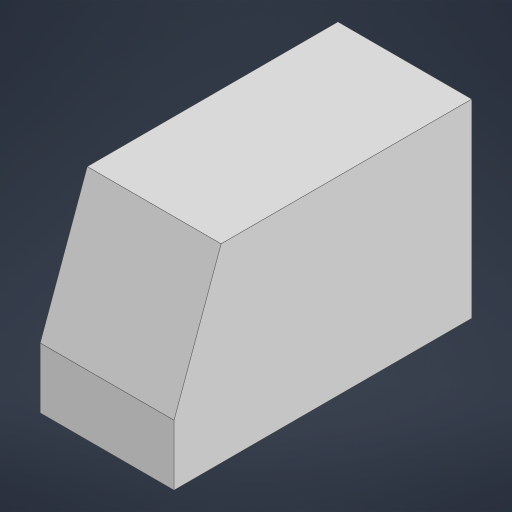
# Autodesk Inventor part: Electronics Case for Bubba
Saved by Autodesk Inventor 2024 (Build 280153000, 153)
## iProperties
Created: 2025-04-03
Part Number: Electronics Case for Bubba
Material: Generic
Document SubType Name: Modeling
Designer: Vincent Larson
Density: 1 g/cm^3
Appearance: Default
Author: Vincent Larson
Autodesk Inventor part; units mm, degrees
ref_plane "YZ Plane" through (0, 0, 0) normal (1, 0, 0) x (0, 1, 0)
ref_plane "XZ Plane" through (0, 0, 0) normal (0, 1, 0) x (-1, 0, 0)
ref_plane "XY Plane" through (0, 0, 0) normal (0, 0, 1) x (1, 0, 0)
sketch "Sketch1" plane through (0, 0, 0) normal (1, 0, 0) x (0, 1, 0)
  line L0 (0, 0) -> (171.45, 0)
  line L1 (171.45, 0) -> (171.45, -271.78)
  line L2 (171.45, -271.78) -> (0, -271.78)
  line L3 (0, -271.78) -> (0, 0)
  line L4 (0, 0) -> (53.34, 0)
  line L5 (53.34, 0) -> (53.34, -271.78)
  line L6 (53.34, 0) -> (171.45, -42.9885)
  line L7 (53.34, 0) -> (179.03, 0) construction
  line L8 (173.99, -274.32) -> (173.99, 2.54)
  line L9 (173.99, 2.54) -> (-2.54, 2.54)
  line L10 (-2.54, 2.54) -> (-2.54, -274.32)
  line L11 (-2.54, -274.32) -> (173.99, -274.32)
  line L12 (54.2087, 2.3868) -> (172.3187, -40.6017)
  line L13 (179.03, -43.0444) -> (43.4558, 6.3006)
  point P0 (53.7879, 2.54)
  point P1 (173.99, -41.21)
  dimension "d0" = 171.45
  dimension "d1" = 271.78
  dimension "d2" = 53.34
  dimension "d3" = 20
  dimension "d4" = 2.54
  dimension "d5" = 2.54
  constraints: 28 end point, 5 parallel, 5 point on line, 3 perpendicular, 2 horizontal, 1 equal length, 3 other
  measures "d0" distance of L1.end L2.end
  measures "d1" distance of L0.end L1.end
  measures "d2" distance of L0.start L4.end
  measures "d3" angle of L6 L7
  measures "d4" distance between parallel lines of L1 L8
  measures "d5" distance between parallel lines of L6 L12
extrude "Extrusion1" add sketch "Sketch1" along normal blind 121.92 contours L3 L2 L1 L12 L13 L8 L11 L10 L9 L0 | L0 L12 L1 L6
sketch "Sketch2" plane through (121.92, 0, 0) normal (1, 0, 0) x (0, 0, -1)
  line L0 (0, 0) -> (0, 53.34) projected
  line L1 (0, 53.34) -> (271.78, 53.34)
  line L2 (271.78, 171.45) -> (271.78, 0) projected
  line L3 (271.78, 55.88) -> (-2.54, 55.88)
  line L4 (-2.54, 55.88) -> (-2.54, 0)
  line L5 (0, 53.34) -> (42.9885, 171.45) projected
  line L6 (5.0738, 67.2802) -> (-1.6206, 48.8875)
  line L7 (271.78, 82.1996) -> (271.78, 27.94)
  point P0 (0.9245, 55.88)
  dimension "d8" = 2.54
  constraints: 10 end point, 4 point on line, 1 collinear, 1 horizontal, 1 other
  measures "d8" distance between parallel lines of L1 L3
extrude "Extrusion2" add sketch "Sketch2" against normal blind 121.92
sketch "Sketch3" plane through (0, -2.54, -274.32) normal (0, 0, -1) x (-1, 0, 0)
  line L0 (0, 0) -> (-121.92, 0) projected
  line L1 (-121.92, 0) -> (0, 0)
  line L2 (-121.92, 55.88) -> (0, 55.88) projected
  line L3 (0, 0) -> (0, 55.88)
  line L4 (0, 55.88) -> (-121.92, 55.88)
  line L5 (0, 58.42) -> (-121.92, 58.42) projected
  line L6 (-121.92, 55.88) -> (-121.92, 0)
  circle A0 centre (-60.96, 27.94) radius 27.94
  line L7 (-83.46, 13.94) -> (-38.46, 13.94)
  line L8 (-38.46, 13.94) -> (-38.46, 41.94)
  line L9 (-38.46, 41.94) -> (-83.46, 41.94)
  line L10 (-83.46, 41.94) -> (-83.46, 13.94)
  line L11 (-83.46, 13.94) -> (-38.46, 41.94) construction
  line L12 (-38.46, 13.94) -> (-83.46, 41.94) construction
  line L13 (-60.9761, 7.94) -> (-60.9439, 7.94)
  line L14 (-60.9439, 47.94) -> (-60.9761, 47.94)
  line L15 (-60.9761, 7.94) -> (-60.9439, 47.94) construction
  line L16 (-60.9439, 7.94) -> (-60.9761, 47.94) construction
  circle A1 centre (-60.96, 47.94) radius 1.8
  circle A2 centre (-60.96, 7.94) radius 1.8
  line L17 (-60.9761, 47.94) -> (-60.9761, 46.1401)
  line L18 (-60.9439, 46.1401) -> (-60.9439, 47.94)
  line L19 (-60.9761, 41.94) -> (-60.9761, 13.94)
  line L20 (-60.9761, 9.7399) -> (-60.9761, 7.94)
  line L21 (-60.9439, 7.94) -> (-60.9439, 9.7399)
  line L22 (-60.9439, 13.94) -> (-60.9439, 41.94)
  point P0 (0, 2.54)
  dimension "d11" = 45
  dimension "d12" = 28
  dimension "d13" = 40
  dimension "d14" = 3.6
  constraints: 40 end point, 13 parallel, 6 midpoint, 6 perpendicular, 4 point on circle, 4 point on line, 3 centre point, 3 horizontal
  measures "d11" distance of L9.end L8.end
  measures "d12" distance of L8.end L7.end
  measures "d13" distance of L14.start L13.end
  measures "d14" diameter of A1
extrude "Extrusion3" cut sketch "Sketch3" against normal blind 121.92 contours L10 L9 L19 L7 | L19 L9 L22 L7 | L22 L9 L8 L7 | L20 A2 L21 L13 | L13 L21 A2 L20 | L18 A1 L17 L14 | L14 L17 A1 L18
sketch "Sketch4" plane through (0, -2.54, -274.32) normal (0, 0, -1) x (-1, 0, 0)
  line L0 (-38.46, 41.94) -> (-38.46, 13.94) projected
  line L1 (-83.46, 13.94) -> (-83.46, 41.94) projected
  line L2 (-38.46, 41.94) -> (-83.46, 41.94)
  line L3 (-83.46, 41.94) -> (-83.46, 13.94)
  line L4 (-83.46, 13.94) -> (-38.46, 13.94)
  line L5 (-38.46, 13.94) -> (-38.46, 41.94)
  line L6 (-86.36, 13.94) -> (-35.56, 13.94)
  line L7 (-35.56, 13.94) -> (-35.56, 41.94)
  line L8 (-35.56, 41.94) -> (-86.36, 41.94)
  line L9 (-86.36, 41.94) -> (-86.36, 13.94)
  line L10 (-86.36, 13.94) -> (-35.56, 41.94) construction
  line L11 (-35.56, 13.94) -> (-86.36, 41.94) construction
  point P0 (0, 2.54)
  point P1 (-60.96, 27.94)
  dimension "d17" = 50.8
  constraints: 20 end point, 4 parallel, 2 horizontal, 2 midpoint, 2 perpendicular
  measures "d17" distance of L8.end L7.end
extrude "Extrusion4" cut sketch "Sketch4" against normal blind 121.92 contours L8 L7 L6 L0 | L1 L6 L9 L8
sketch "Sketch5" plane through (121.92, 0, 0) normal (1, 0, 0) x (0, 0, -1)
  line L0 (271.78, 53.34) -> (271.78, 0) projected
  line L1 (271.78, 53.34) -> (246.38, 53.34)
  line L2 (271.78, 53.34) -> (0, 53.34) projected
  line L3 (246.38, 53.34) -> (246.38, 43.18)
  line L4 (246.38, 43.18) -> (272.1958, 43.18)
  line L5 (246.38, 43.18) -> (226.8063, 53.34)
  line L6 (226.8063, 53.34) -> (209.4202, 62.3644)
  line L7 (245.2098, 40.9256) -> (225.6361, 51.0856)
  line L8 (225.6361, 51.0856) -> (208.25, 60.1101)
  line L9 (246.38, 40.64) -> (272.1958, 40.64)
  line L10 (239.3965, 43.9431) -> (259.2879, 33.6182)
  line L11 (267.1647, 40.64) -> (232.6379, 40.64)
  point P0 (0, 0)
  point P1 (245.7601, 40.64)
  point P2 (271.78, 40.64)
  point P3 (271.78, 43.18)
  point P4 (221.2929, 53.34)
  dimension "d20" = 25.4
  dimension "d21" = 10.16
  dimension "d22" = 2.54
  dimension "d23" = 2.54
  constraints: 20 end point, 7 point on line, 1 parallel, 1 perpendicular, 1 vertical, 1 other
  measures "d20" distance of L0.start L1.end
  measures "d21" distance of L1.end L3.end
  measures "d22" distance between parallel lines of L5 L7
  measures "d23" distance between parallel lines of L4 L9
extrude "Extrusion5" add sketch "Sketch5" against normal blind 121.92 contours L0 L9 L11 L10 L7 L8 L2 L5 L4
sketch "Sketch6" plane through (0, 0, 0) normal (-1, 0, 0) x (0, 0, 1)
  line L0 (-226.8063, 53.34) -> (-246.38, 43.18) projected
  line L1 (-233.7398, 49.741) -> (-197.786, 68.4033)
  line L2 (-197.786, 68.4033) -> (-271.78, 69.3117)
  line L3 (-271.78, 171.45) -> (-271.78, 55.88) projected
  line L4 (-271.78, 69.3117) -> (-271.78, 47.3341)
  line L5 (-271.78, 53.34) -> (-271.78, 43.18) projected
  line L6 (-271.78, 47.3341) -> (-233.7398, 49.741)
  point P0 (0, 0)
  constraints: 8 end point, 3 point on line, 1 collinear
extrude "Extrusion6" cut sketch "Sketch6" against normal blind 121.92
sketch "Sketch7" plane through (121.92, 0, 0) normal (1, 0, 0) x (0, 0, -1)
  line L0 (-2.54, -2.54) -> (274.32, -2.54) projected
  line L1 (274.32, 173.99) -> (41.21, 173.99) projected
  line L2 (-2.54, -2.54) -> (274.32, -2.54)
  line L3 (274.32, -2.54) -> (274.32, 173.99)
  line L4 (274.32, 173.99) -> (-2.54, 173.99)
  line L5 (-2.54, 173.99) -> (-2.54, -2.54)
  line L6 (41.21, 173.99) -> (-2.54, 53.7879) projected
  line L7 (41.21, 173.99) -> (-2.54, 53.7879)
  point P0 (0, 0)
  constraints: 10 end point, 3 equal length, 1 horizontal, 1 perpendicular
extrude "Extrusion7" add sketch "Sketch7" along normal blind 2.54 contours L5 L6 L1 L3 L0
sketch "Sketch8" plane through (0, -2.54, -274.32) normal (0, 0, -1) x (-1, 0, 0)
  line L0 (0, 173.99) -> (-121.92, 173.99) projected
  line L1 (-121.92, 173.99) -> (0, 173.99)
  line L2 (0, 173.99) -> (0, 52.07)
  line L3 (0, 52.07) -> (-121.92, 52.07)
  line L4 (-121.92, 52.07) -> (-121.92, 173.99)
  circle A0 centre (-60.96, 113.03) radius 57.15
  point P0 (0, 2.54)
  dimension "d30" = 121.92
  dimension "d31" = 114.3
  constraints: 8 end point, 2 parallel, 1 centre point, 1 horizontal, 1 perpendicular
  measures "d30" distance of L1.end L2.end
  measures "d31" diameter of A0
extrude "Extrusion8" cut sketch "Sketch8" against normal blind 25.4 contours A0
body "Solid1"
